Autodesk Fusion 360 part; units mm, degrees
note: some values were not read from the file. Set by a fixed rule: which sketch regions a step uses.
(part 3 of 3)
  circle A902 centre (-15.0186, -206.3325) radius 0.5023
  circle A903 centre (-15.0186, -209.9835) radius 0.5023
  circle A904 centre (-15.0186, -213.6344) radius 0.5023
  circle A905 centre (-15.0186, -217.2853) radius 0.5023
  circle A906 centre (-15.0186, -220.9363) radius 0.5023
  circle A907 centre (-15.0186, -224.5872) radius 0.5023
extrude "Estrusione56" cut sketch "Schizzo100" against normal blind 1 contours A0 | A1 | A2 | A3 | A4 | A5 | A6 | A7 | A8 | A9 | A10 | A11 | A12 | A13 | A14 | A15 | A16 | A17 | A18 | A19 | A20 | A21 | A22 | A23 | A24 | A25 | A26 | A27 | A28 | A29 | A30 | A31 | A32 | A33 | A34 | A35 | A36 | A37 | A38 | A39 | A40 | A41 | A42 | A43 | A44 | A45 | A46 | A47 | A48 | A49 | A50 | A51 | A52 | A53 | A54 | A55 | A56 | A57 | A58 | A59 | A60 | A61 | A62 | A63 | A64 | A65 | A66 | A67 | A68 | A69 | A70 | A71 | A72 | A73 | A74 | A75 | A76 | A77 | A78 | A79 | A80 | A81 | A82 | A83 | A84 | A85 | A86 | A87 | A88 | A89 | A90 | A91 | A92 | A93 | A94 | A95 | A96 | A97 | A98 | A99 | A100 | A101 | A102 | A103 | A104 | A105 | A106 | A107 | A108 | A109 | A110 | A111 | A112 | A113 | A114 | A115 | A116 | A117 | A118 | A119 | A120 | A121 | A122 | A123 | A124 | A125 | A126 | A127 | A128 | A129 | A130 | A131 | A132 | A133 | A134 | A135 | A136 | A137 | A138 | A139 | A140 | A141 | A142 | A143 | A144 | A145 | A146 | A147 | A148 | A149 | A150 | A151 | A152 | A153 | A154 | A155 | A156 | A157 | A158 | A159 | A160 | A161 | A162 | A163 | A164 | A165 | A166 | A167 | A168 | A169 | A170 | A171 | A172 | A173 | A174 | A175 | A176 | A177 | A178 | A179 | A180 | A181 | A182 | A183 | A184 | A185 | A186 | A187 | A188 | A189 | A190 | A191 | A192 | A193 | A194 | A195 | A196 | A197 | A198 | A199 | A200 | A201 | A202 | A203 | A204 | A205 | A206 | A207 | A208 | A209 | A210 | A211 | A212 | A213 | A214 | A215 | A216 | A217 | A218 | A219 | A220 | A221 | A222 | A223 | A224 | A225 | A226 | A227 | A228 | A229 | A230 | A231 | A232 | A233 | A234 | A235 | A236 | A237 | A238 | A239 | A240 | A241 | A242 | A243 | A244 | A245 | A246 | A247 | A248 | A249 | A250 | A251 | A252 | A253 | A254 | A255 | A256 | A257 | A258 | A259 | A260 | A261 | A262 | A263 | A264 | A265 | A266 | A267 | A268 | A269 | A270 | A271 | A272 | A273 | A274 | A275 | A276 | A277 | A278 | A279 | A280 | A281 | A282 | A283 | A284 | A285 | A286 | A287 | A288 | A289 | A290 | A291 | A292 | A293 | A294 | A295 | A296 | A297 | A298 | A299 | A300 | A301 | A302 | A303 | A304 | A305 | A306 | A307 | A308 | A309 | A310 | A311 | A312 | A313 | A314 | A315 | A316 | A317 | A318 | A319 | A320 | A321 | A322 | A323 | A324 | A325 | A326 | A327 | A328 | A329 | A330 | A331 | A332 | A333 | A334 | A335 | A336 | A337 | A338 | A339 | A340 | A341 | A342 | A343 | A344 | A345 | A346 | A347 | A348 | A349 | A350 | A351 | A352 | A353 | A354 | A355 | A356 | A357 | A358 | A359 | A360 | A361 | A362 | A363 | A364 | A365 | A366 | A367 | A368 | A369 | A370 | A371 | A372 | A373 | A374 | A375 | A376 | A377 | A378 | A379 | A380 | A381 | A382 | A383 | A384 | A385 | A386 | A387 | A388 | A389 | A390 | A391 | A392 | A393 | A394 | A395 | A396 | A397 | A398 | A399 | A400 | A401 | A402 | A403 | A404 | A405 | A406 | A407 | A408 | A409 | A410 | A411 | A412 | A413 | A414 | A415 | A416 | A417 | A418 | A419 | A420 | A421 | A422 | A423 | A424 | A425 | A426 | A427 | A428 | A429 | A430 | A431 | A432 | A433 | A434 | A435 | A436 | A437 | A438 | A439 | A440 | A441 | A442 | A443 | A444 | A445 | A446 | A447 | A448 | A449 | A450 | A451 | A452 | A453 | A454 | A455 | A456 | A457 | A458 | A459 | A460 | A461 | A462 | A463 | A464 | A465 | A466 | A467 | A468 | A469 | A470 | A471 | A472 | A473 | A474 | A475 | A476 | A477 | A478 | A479 | A480 | A481 | A482 | A483 | A484 | A485 | A486 | A487 | A488 | A489 | A490 | A491 | A492 | A493 | A494 | A495 | A496 | A497 | A498 | A499 | A500 | A501 | A502 | A503 | A504 | A505 | A506 | A507 | A508 | A509 | A510 | A511 | A512 | A513 | A514 | A515 | A516 | A517 | A518 | A519 | A520 | A521 | A522 | A523 | A524 | A525 | A526 | A527 | A528 | A529 | A530 | A531 | A532 | A533 | A534 | A535 | A536 | A537 | A538 | A539 | A540 | A541 | A542 | A543 | A544 | A545 | A546 | A547 | A548 | A549 | A550 | A551 | A552 | A553 | A554 | A555 | A556 | A557 | A558 | A559 | A560 | A561 | A562 | A563 | A564 | A565 | A566 | A567 | A568 | A569 | A570 | A571 | A572 | A573 | A574 | A575 | A576 | A577 | A578 | A579 | A580 | A581 | A582 | A583 | A584 | A585 | A586 | A587 | A588 | A589 | A590 | A591 | A592 | A593 | A594 | A595 | A596 | A597 | A598 | A599 | A600 | A601 | A602 | A603 | A604 | A605 | A606 | A607 | A608 | A609 | A610 | A611 | A612 | A613 | A614 | A615 | A616 | A617 | A618 | A619 | A620 | A621 | A622 | A623 | A624 | A625 | A626 | A627 | A628 | A629 | A630 | A631 | A632 | A633 | A634 | A635 | A636 | A637 | A638 | A639 | A640 | A641 | A642 | A643 | A644 | A645 | A646 | A647 | A648 | A649 | A650 | A651 | A652 | A653 | A654 | A655 | A656 | A657 | A658 | A659 | A660 | A661 | A662 | A663 | A664 | A665 | A666 | A667 | A668 | A669 | A670 | A671 | A672 | A673 | A674 | A675 | A676 | A677 | A678 | A679 | A680 | A681 | A682 | A683 | A684 | A685 | A686 | A687 | A688 | A689 | A690 | A691 | A692 | A693 | A694 | A695 | A696 | A697 | A698 | A699 | A700 | A701 | A702 | A703 | A704 | A705 | A706 | A707 | A708 | A709 | A710 | A711 | A712 | A713 | A714 | A715 | A716 | A717 | A718 | A719 | A720 | A721 | A722 | A723 | A724 | A725 | A726 | A727 | A728 | A729 | A730 | A731 | A732 | A733 | A734 | A735 | A736 | A737 | A738 | A739 | A740 | A741 | A742 | A743 | A744 | A745 | A746 | A747 | A748 | A749 | A750 | A751 | A752 | A753 | A754 | A755 | A756 | A757 | A758 | A759 | A760 | A761 | A762 | A763 | A764 | A765 | A766 | A767 | A768 | A769 | A770 | A771 | A772 | A773 | A774 | A775 | A776 | A777 | A778 | A779 | A780 | A781 | A782 | A783 | A784 | A785 | A786 | A787 | A788 | A789 | A790 | A791 | A792 | A793 | A794 | A795 | A796 | A797 | A798 | A799 | A800 | A801 | A802 | A803 | A804 | A805 | A806 | A807 | A808 | A809 | A810 | A811 | A812 | A813 | A814 | A815 | A816 | A817 | A818 | A819 | A820 | A821 | A822 | A823 | A824 | A825 | A826 | A827 | A828 | A829 | A830 | A831 | A832 | A833 | A834 | A835 | A836 | A837 | A838 | A839 | A840 | A841 | A842 | A843 | A844 | A845 | A846 | A847 | A848 | A849 | A850 | A851 | A852 | A853 | A854 | A855 | A856 | A857 | A858 | A859 | A860 | A861 | A862 | A863 | A864 | A865 | A866 | A867 | A868 | A869 | A870 | A871 | A872 | A873 | A874 | A875 | A876 | A877 | A878 | A879 | A880 | A881 | A882 | A883 | A884 | A885 | A886 | A887 | A888 | A889 | A890 | A891 | A892 | A893 | A894 | A895 | A896 | A897 | A898 | A899 | A900 | A901 | A902 | A903 | A904 | A905 | A906 | A907 picked at (15.0787, -5.3673) picked at (15.0787, -9.0183) picked at (15.0879, -12.8411) picked at (14.9196, -16.6361) picked at (14.8948, -20.2907) picked at (14.7587, -23.8997) picked at (14.8948, -27.5926) picked at (15.0731, -30.9982) picked at (15.3096, -34.6996) picked at (15.0912, -38.254) picked at (15.3096, -42.0014) picked at (15.3096, -45.6524) picked at (15.3096, -49.3033) picked at (15.3096, -52.9542) picked at (14.8814, -56.9112) picked at (15.3096, -60.2561) picked at (14.8709, -63.7829) picked at (14.6953, -67.6913) picked at (14.6953, -71.3423) picked at (14.6953, -74.9932) picked at (14.6953, -78.6441) picked at (15.0397, -82.3458) picked at (14.6953, -85.946) picked at (14.8598, -89.1907) picked at (14.6953, -93.2479) picked at (14.6953, -96.8988) picked at (14.6953, -100.5497) picked at (14.6953, -104.2007) picked at (15.0397, -107.9023) picked at (14.6953, -111.5026) picked at (14.7771, -115.1901) picked at (15.0397, -118.8551) picked at (15.0397, -122.506) picked at (15.0397, -126.157) picked at (15.1827, -129.532) picked at (15.1142, -133.1688) picked at (15.1142, -136.8198) picked at (15.0787, -140.4031) picked at (15.0787, -144.0541) picked at (15.0787, -147.705) picked at (15.1827, -151.4376) picked at (15.1827, -155.0886) picked at (15.1827, -158.7395) picked at (15.1827, -162.3904) picked at (15.1827, -166.0414) picked at (15.1827, -169.6923) picked at (15.1827, -173.3432) picked at (15.1827, -176.9942) picked at (15.1142, -180.631) picked at (15.1142, -184.2819) picked at (15.1142, -187.9329) picked at (15.0787, -191.5162) picked at (15.0787, -195.1672) picked at (15.0787, -198.8181) picked at (15.1827, -202.5507) picked at (15.1827, -206.2016) picked at (15.1827, -209.8526) picked at (15.1827, -213.5035) picked at (15.1827, -217.1544) picked at (15.1827, -220.8054) picked at (15.1827, -224.4563) picked at (13.2695, -7.1766) picked at (13.0358, -10.727) picked at (13.0358, -14.378) picked at (13.0575, -18.5125) picked at (13.0575, -22.1634) picked at (13.0856, -25.7509) picked at (13.0575, -29.4653) picked at (13.5004, -32.8578) picked at (13.2555, -36.4028) picked at (13.2555, -40.0538) picked at (13.2555, -43.7047) picked at (13.2555, -47.3556) picked at (13.5004, -51.1125) picked at (13.2555, -54.6575) picked at (13.0173, -58.3225) picked at (13.2555, -61.9594) picked at (13.1095, -65.5921) picked at (13.1095, -69.243) picked at (13.1095, -72.894) picked at (12.8861, -76.8024) picked at (13.1095, -80.1958) picked at (13.0505, -83.698) picked at (13.1095, -87.4977) picked at (13.1095, -91.1486) picked at (13.1095, -94.7996) picked at (13.1095, -98.4505) picked at (12.8861, -102.359) picked at (13.1095, -105.7524) picked at (13.0505, -109.2546) picked at (13.1095, -113.0542) picked at (13.1095, -116.7052) picked at (12.8861, -120.6137) picked at (12.8861, -124.2646) picked at (13.0084, -127.9155) picked at (13.2851, -131.3778) picked at (13.2851, -135.0288) picked at (13.305, -138.629) picked at (13.305, -142.2799) picked at (13.305, -145.9309) picked at (12.9495, -149.8407) picked at (12.9495, -153.4916) picked at (12.9495, -157.1426) picked at (12.9495, -160.7935) picked at (12.9495, -164.4444) picked at (12.9495, -168.0954) picked at (12.9495, -171.7463) picked at (12.9495, -175.3972) picked at (13.2851, -178.84) picked at (13.2851, -182.4909) picked at (13.2851, -186.1418) picked at (13.305, -189.7421) picked at (13.305, -193.393) picked at (12.9495, -197.3028) picked at (12.9495, -200.9538) picked at (12.9495, -204.6047) picked at (12.9495, -208.2557) picked at (12.9495, -211.9066) picked at (12.9495, -215.5575) picked at (12.9495, -219.2085) picked at (12.9495, -222.8594) picked at (10.7966, -5.3673) picked at (10.7966, -9.0183) picked at (10.8058, -12.8411) picked at (10.6375, -16.6361) picked at (10.6127, -20.2907) picked at (10.4766, -23.8997) picked at (10.6127, -27.5926) picked at (10.7911, -30.9982) picked at (11.0276, -34.6996) picked at (10.8091, -38.254) picked at (11.0276, -42.0014) picked at (11.0276, -45.6524) picked at (11.0276, -49.3033) picked at (11.0276, -52.9542) picked at (10.5993, -56.9112) picked at (11.0276, -60.2561) picked at (10.5888, -63.7829) picked at (10.4132, -67.6913) picked at (10.4132, -71.3423) picked at (10.4132, -74.9932) picked at (10.4132, -78.6441) picked at (10.7576, -82.3458) picked at (10.4132, -85.946) picked at (10.5777, -89.1907) picked at (10.4132, -93.2479) picked at (10.4132, -96.8988) picked at (10.4132, -100.5497) picked at (10.4132, -104.2007) picked at (10.7576, -107.9023) picked at (10.4132, -111.5026) picked at (10.495, -115.1901) picked at (10.7576, -118.8551) picked at (10.7576, -122.506) picked at (10.7576, -126.157) picked at (10.9006, -129.532) picked at (10.8321, -133.1688) picked at (10.8321, -136.8198) picked at (10.7966, -140.4031) picked at (10.7966, -144.0541) picked at (10.7966, -147.705) picked at (10.9006, -151.4376) picked at (10.9006, -155.0886) picked at (10.9006, -158.7395) picked at (10.9006, -162.3904) picked at (10.9006, -166.0414) picked at (10.9006, -169.6923) picked at (10.9006, -173.3432) picked at (10.9006, -176.9942) picked at (10.8321, -180.631) picked at (10.8321, -184.2819) picked at (10.8321, -187.9329) picked at (10.7966, -191.5162) picked at (10.7966, -195.1672) picked at (10.7966, -198.8181) picked at (10.9006, -202.5507) picked at (10.9006, -206.2016) picked at (10.9006, -209.8526) picked at (10.9006, -213.5035) picked at (10.9006, -217.1544) picked at (10.9006, -220.8054) picked at (10.9006, -224.4563) picked at (8.9874, -7.1766) picked at (8.9874, -10.8275) picked at (8.9874, -14.4784) picked at (8.8366, -18.5784) picked at (8.8366, -22.2293) picked at (8.8035, -25.7509) picked at (8.8366, -29.5312) picked at (8.7559, -33.0419) picked at (8.9258, -36.7037) picked at (8.9258, -40.3546) picked at (8.9258, -44.0056) picked at (8.9258, -47.6565) picked at (8.7559, -51.2966) picked at (8.9258, -54.9584) picked at (8.7353, -58.3225) picked at (8.9258, -62.2602) picked at (9.0124, -65.6414) picked at (9.0124, -69.2924) picked at (9.0124, -72.9433) picked at (8.604, -76.8024) picked at (9.0124, -80.2452) picked at (8.7684, -83.698) picked at (9.0124, -87.547) picked at (9.0124, -91.198) picked at (9.0124, -94.8489) picked at (9.0124, -98.4998) picked at (8.604, -102.359) picked at (9.0124, -105.8017) picked at (8.7684, -109.2546) picked at (9.0124, -113.1036) picked at (9.0124, -116.7545) picked at (8.604, -120.6137) picked at (8.604, -124.2646) picked at (8.7263, -127.9155) picked at (9.003, -131.3778) picked at (9.003, -135.0288) picked at (9.0229, -138.629) picked at (9.0229, -142.2799) picked at (9.0229, -145.9309) picked at (8.6674, -149.8407) picked at (8.6674, -153.4916) picked at (8.6674, -157.1426) picked at (8.6674, -160.7935) picked at (8.6674, -164.4444) picked at (8.6674, -168.0954) picked at (8.6674, -171.7463) picked at (8.6674, -175.3972) picked at (9.003, -178.84) picked at (9.003, -182.4909) picked at (9.003, -186.1418) picked at (9.0229, -189.7421) picked at (9.0229, -193.393) picked at (8.6674, -197.3028) picked at (8.6674, -200.9538) picked at (8.6674, -204.6047) picked at (8.6674, -208.2557) picked at (8.6674, -211.9066) picked at (8.6674, -215.5575) picked at (8.6674, -219.2085) picked at (8.6674, -222.8594) picked at (6.5499, -5.5067) picked at (6.5482, -9.1837) picked at (6.5501, -12.955) picked at (6.3554, -16.6361) picked at (6.3306, -20.2907) picked at (6.5891, -23.6719) picked at (6.3306, -27.5926) picked at (6.5201, -31.0481) picked at (6.7455, -34.7777) picked at (6.5427, -38.4622) picked at (6.7455, -42.0795) picked at (6.7455, -45.7305) picked at (6.7455, -49.3814) picked at (6.7455, -53.0323) picked at (6.5482, -56.6459) picked at (6.7455, -60.3342) picked at (6.453, -64.1019) picked at (6.6525, -67.5027) picked at (6.6525, -71.1536) picked at (6.6525, -74.8046) picked at (6.6525, -78.4555) picked at (6.3081, -82.0558) picked at (6.6525, -85.7574) picked at (6.2956, -89.1907) picked at (6.6525, -93.0592) picked at (6.6525, -96.7102) picked at (6.6525, -100.3611) picked at (6.6525, -104.0121) picked at (6.3081, -107.6123) picked at (6.6525, -111.3139) picked at (6.5891, -114.9453) picked at (6.3081, -118.5651) picked at (6.3081, -122.216) picked at (6.3081, -125.867) picked at (6.1651, -129.7938) picked at (6.2336, -133.4588) picked at (6.2336, -137.1098) picked at (6.2691, -140.8283) picked at (6.2691, -144.4792) picked at (6.2691, -148.1302) picked at (6.1651, -151.6994) picked at (6.6185, -155.0886) picked at (6.1651, -159.0013) picked at (6.1651, -162.6522) picked at (6.1651, -166.3032) picked at (6.6185, -169.6923) picked at (6.1651, -173.605) picked at (6.6185, -176.9942) picked at (6.2336, -180.921) picked at (6.2336, -184.5719) picked at (6.2336, -188.2229) picked at (6.2691, -191.9414) picked at (6.2691, -195.5923) picked at (6.2691, -199.2433) picked at (6.1651, -202.8125) picked at (6.1651, -206.4634) picked at (6.1651, -210.1144) picked at (6.1651, -213.7653) picked at (6.1651, -217.4163) picked at (6.1651, -221.0672) picked at (6.1651, -224.7181) picked at (4.7142, -7.5905) picked at (4.5486, -11.2664) picked at (4.5486, -14.9173) picked at (4.5361, -18.5466) picked at (4.5361, -22.1975) picked at (4.4728, -25.4281) picked at (4.5361, -29.4994) picked at (4.4532, -33.0278) picked at (4.4026, -36.3809) picked at (4.6913, -40.0538) picked at (4.4026, -43.6827) picked at (4.6913, -47.3556) picked at (4.4532, -51.2825) picked at (4.6913, -54.6575) picked at (4.5701, -58.3586) picked at (4.6913, -61.9594) picked at (4.4348, -65.8692) picked at (4.4348, -69.5201) picked at (4.4348, -73.1711) picked at (4.8433, -76.6138) picked at (4.4348, -80.4729) picked at (4.4864, -83.698) picked at (4.4348, -87.7748) picked at (4.4348, -91.4257) picked at (4.4348, -95.0767) picked at (4.4348, -98.7276) picked at (4.8433, -102.1703) picked at (4.4348, -106.0295) picked at (4.4864, -109.2546) picked at (4.4348, -113.3313) picked at (4.4348, -116.9823) picked at (4.8433, -120.425) picked at (4.8433, -124.076) picked at (4.75, -128.0098) picked at (4.4442, -131.5665) picked at (4.4442, -135.2174) picked at (4.4244, -138.919) picked at (4.4244, -142.5699) picked at (4.4244, -146.2209) picked at (4.7798, -149.6129) picked at (4.7798, -153.2639) picked at (4.7798, -156.9148) picked at (4.7798, -160.5657) picked at (4.7798, -164.2167) picked at (4.7798, -167.8676) picked at (4.7798, -171.5185) picked at (4.7798, -175.1695) picked at (4.4442, -179.0286) picked at (4.4442, -182.6795) picked at (4.4442, -186.3305) picked at (4.4244, -190.0321) picked at (4.4244, -193.683) picked at (4.7798, -197.0751) picked at (4.7798, -200.726) picked at (4.7798, -204.377) picked at (4.7798, -208.0279) picked at (4.7798, -211.6788) picked at (4.7798, -215.3298) picked at (4.7798, -218.9807) picked at (4.7798, -222.6316) picked at (2.0725, -5.6944) picked at (2.2325, -9.3799) picked at (2.2697, -12.7836) picked at (2.0972, -16.3244) picked at (2.3548, -20.021) picked at (2.3548, -23.6719) picked at (2.3548, -27.3229) picked at (2.0053, -30.9908) picked at (2.001, -34.8836) picked at (2.2499, -38.3202) picked at (2.001, -42.1855) picked at (2.001, -45.8364) picked at (1.9091, -49.4952) picked at (1.9091, -53.1461) picked at (1.9464, -56.5499) picked at (2.001, -60.4401) picked at (2.0486, -63.7902) picked at (2.3704, -67.5027) picked at (2.3704, -71.1536) picked at (2.3704, -74.8046) picked at (2.3704, -78.4555) picked at (2.026, -82.0558) picked at (2.3704, -85.7574) picked at (2.0135, -89.1907) picked at (2.3704, -93.0592) picked at (2.3704, -96.7102) picked at (2.3704, -100.3611) picked at (2.3704, -104.0121) picked at (2.026, -107.6123) picked at (2.3704, -111.3139) picked at (2.307, -114.9453) picked at (2.026, -118.5651) picked at (2.026, -122.216) picked at (2.026, -125.867) picked at (2.3365, -129.532) picked at (2.268, -133.1688) picked at (2.268, -136.8198) picked at (2.2325, -140.4031) picked at (2.2325, -144.0541) picked at (2.2325, -147.705) picked at (2.3365, -151.4376) picked at (2.3365, -155.0886) picked at (2.3365, -158.7395) picked at (2.3365, -162.3904) picked at (2.3365, -166.0414) picked at (2.3365, -169.6923) picked at (2.3365, -173.3432) picked at (2.3365, -176.9942) picked at (2.268, -180.631) picked at (2.268, -184.2819) picked at (2.268, -187.9329) picked at (2.2325, -191.5162) picked at (2.2325, -195.1672) picked at (2.2325, -198.8181) picked at (2.3365, -202.5507) picked at (2.3365, -206.2016) picked at (2.3365, -209.8526) picked at (2.3365, -213.5035) picked at (2.3365, -217.1544) picked at (2.3365, -220.8054) picked at (2.3365, -224.4563) picked at (0.2783, -7.2156) picked at (0.2632, -10.8281) picked at (0.2632, -14.479) picked at (0.1456, -18.1262) picked at (0.1456, -21.7771) picked at (0.1478, -25.6427) picked at (0.1456, -29.079) picked at (0.4388, -32.8525) picked at (0.1961, -36.4169) picked at (0.1961, -40.0679) picked at (0.1961, -43.7188) picked at (0.1961, -47.3697) picked at (0.4388, -51.1072) picked at (0.1961, -54.6716) picked at (0.4588, -58.5754) picked at (0.1961, -61.9735) picked at (0.2043, -65.4434) picked at (0.2043, -69.0943) picked at (0.2043, -72.7452) picked at (0.4977, -76.5942) picked at (0.2043, -80.0471) picked at (0.4049, -83.8791) picked at (0.2043, -87.349) picked at (0.2043, -90.9999) picked at (0.2043, -94.6508) picked at (0.2043, -98.3018) picked at (0.4977, -102.1508) picked at (0.2043, -105.6036) picked at (0.4049, -109.4356) picked at (0.2043, -112.9055) picked at (0.2043, -116.5564) picked at (0.4977, -120.4055) picked at (0.4977, -124.0564) picked at (0.0793, -127.9425) picked at (0.4977, -131.3583) picked at (0.4977, -135.0092) picked at (0.5272, -138.6431) picked at (0.5272, -142.294) picked at (0.5272, -145.945) picked at (-0.0178, -149.7995) picked at (-0.0178, -153.4504) picked at (-0.0178, -157.1013) picked at (-0.0178, -160.7523) picked at (-0.0178, -164.4032) picked at (-0.0178, -168.0541) picked at (-0.0178, -171.7051) picked at (-0.0178, -175.356) picked at (0.4977, -178.8204) picked at (0.4977, -182.4713) picked at (0.4977, -186.1223) picked at (0.5272, -189.7562) picked at (0.5272, -193.4071) picked at (-0.0178, -197.2616) picked at (-0.0178, -200.9125) picked at (-0.0178, -204.5635) picked at (-0.0178, -208.2144) picked at (-0.0178, -211.8654) picked at (-0.0178, -215.5163) picked at (-0.0178, -219.1672) picked at (-0.0178, -222.8182) picked at (-2.2096, -5.6944) picked at (-2.1913, -9.0358) picked at (-2.0141, -12.955) picked at (-2.1849, -16.3244) picked at (-1.9273, -20.021) picked at (-1.9273, -23.6719) picked at (-1.9273, -27.3229) picked at (-2.2768, -30.9908) picked at (-2.0636, -34.5936) picked at (-2.3379, -38.2259) picked at (-2.0636, -41.8955) picked at (-2.0636, -45.5464) picked at (-2.373, -49.4952) picked at (-2.373, -53.1461) picked at (-2.2561, -56.7892) picked at (-2.0636, -60.1502) picked at (-2.2335, -63.7902) picked at (-2.4556, -67.6805) picked at (-2.4556, -71.3314) picked at (-2.4556, -74.9823) picked at (-2.4556, -78.6333) picked at (-2.2561, -82.0558) picked at (-2.4556, -85.9352) picked at (-2.0068, -89.7162) picked at (-2.4556, -93.237) picked at (-2.4556, -96.888) picked at (-2.4556, -100.5389) picked at (-2.4556, -104.1898) picked at (-2.2561, -107.6123) picked at (-2.4556, -111.4917) picked at (-1.9751, -114.9453) picked at (-2.2561, -118.5651) picked at (-2.2561, -122.216) picked at (-2.2561, -125.867) picked at (-1.9456, -129.532) picked at (-2.0141, -133.1688) picked at (-2.0141, -136.8198) picked at (-2.2951, -140.8283) picked at (-2.2951, -144.4792) picked at (-2.2951, -148.1302) picked at (-1.9456, -151.4376) picked at (-1.9456, -155.0886) picked at (-1.9456, -158.7395) picked at (-1.9456, -162.3904) picked at (-1.9456, -166.0414) picked at (-1.9456, -169.6923) picked at (-1.9456, -173.3432) picked at (-1.9456, -176.9942) picked at (-2.0141, -180.631) picked at (-2.0141, -184.2819) picked at (-2.0141, -187.9329) picked at (-2.2951, -191.9414) picked at (-2.2951, -195.5923) picked at (-2.2951, -199.2433) picked at (-1.9456, -202.5507) picked at (-1.9456, -206.2016) picked at (-1.9456, -209.8526) picked at (-1.9456, -213.5035) picked at (-1.9456, -217.1544) picked at (-1.9456, -220.8054) picked at (-1.9456, -224.4563) picked at (-3.8441, -7.5019) picked at (-4.1232, -11.0577) picked at (-4.1232, -14.7086) picked at (-4.0914, -18.1262) picked at (-4.0914, -21.7771) picked at (-3.8589, -25.743) picked at (-4.0914, -29.079) picked at (-3.8307, -32.9695) picked at (-4.1822, -36.7007) picked at (-4.0903, -40.3438) picked at (-4.1822, -44.0026) picked at (-4.0903, -47.6456) picked at (-3.8307, -51.2242) picked at (-4.0903, -54.9475) picked at (-3.8451, -58.3342) picked at (-4.0903, -62.2494) picked at (-4.0914, -65.5884) picked at (-4.0914, -69.2393) picked at (-4.0914, -72.8902) picked at (-4.0653, -76.5631) picked at (-4.0914, -80.1921) picked at (-3.7843, -83.8961) picked at (-4.0914, -87.494) picked at (-4.0914, -91.1449) picked at (-4.0914, -94.7958) picked at (-4.0914, -98.4468) picked at (-4.0653, -102.1197) picked at (-4.0914, -105.7486) picked at (-3.7843, -109.4527) picked at (-4.0914, -113.0505) picked at (-4.0914, -116.7014) picked at (-4.0653, -120.3743) picked at (-4.0653, -124.0253) picked at (-3.9941, -127.7995) picked at (-3.8234, -131.3271) picked at (-3.8234, -134.9781) picked at (-4.1043, -138.9866) picked at (-4.1043, -142.6375) picked at (-4.1043, -146.2885) picked at (-4.2083, -149.8577) picked at (-4.2083, -153.5087) picked at (-4.2083, -157.1596) picked at (-4.2083, -160.8105) picked at (-4.2083, -164.4615) picked at (-4.2083, -168.1124) picked at (-4.2083, -171.7633) picked at (-4.2083, -175.4143) picked at (-3.8234, -178.7893) picked at (-3.8234, -182.4402) picked at (-3.8234, -186.0912) picked at (-4.1043, -190.0997) picked at (-4.1043, -193.7506) picked at (-4.2083, -197.3199) picked at (-4.2083, -200.9708) picked at (-4.2083, -204.6217) picked at (-4.2083, -208.2727) picked at (-4.2083, -211.9236) picked at (-4.2083, -215.5745) picked at (-4.2083, -219.2255) picked at (-4.2083, -222.8764) picked at (-6.2963, -5.5067) picked at (-6.298, -9.1837) picked at (-6.2962, -12.955) picked at (-6.4909, -16.6361) picked at (-6.5156, -20.2907) picked at (-6.2572, -23.6719) picked at (-6.5156, -27.5926) picked at (-6.3261, -31.0481) picked at (-6.1008, -34.7777) picked at (-6.3036, -38.4622) picked at (-6.1008, -42.0795) picked at (-6.1008, -45.7305) picked at (-6.1008, -49.3814) picked at (-6.1008, -53.0323) picked at (-6.298, -56.6459) picked at (-6.1008, -60.3342) picked at (-6.3933, -64.1019) picked at (-6.1938, -67.5027) picked at (-6.1938, -71.1536) picked at (-6.1938, -74.8046) picked at (-6.1938, -78.4555) picked at (-6.5382, -82.0558) picked at (-6.1938, -85.7574) picked at (-6.5507, -89.1907) picked at (-6.1938, -93.0592) picked at (-6.1938, -96.7102) picked at (-6.1938, -100.3611) picked at (-6.1938, -104.0121) picked at (-6.5382, -107.6123) picked at (-6.1938, -111.3139) picked at (-6.2572, -114.9453) picked at (-6.5382, -118.5651) picked at (-6.5382, -122.216) picked at (-6.5382, -125.867) picked at (-6.6812, -129.7938) picked at (-6.6127, -133.4588) picked at (-6.6127, -137.1098) picked at (-6.5772, -140.8283) picked at (-6.5772, -144.4792) picked at (-6.5772, -148.1302) picked at (-6.6812, -151.6994) picked at (-6.2277, -155.0886) picked at (-6.6812, -159.0013) picked at (-6.6812, -162.6522) picked at (-6.6812, -166.3032) picked at (-6.2277, -169.6923) picked at (-6.6812, -173.605) picked at (-6.2277, -176.9942) picked at (-6.6127, -180.921) picked at (-6.6127, -184.5719) picked at (-6.6127, -188.2229) picked at (-6.5772, -191.9414) picked at (-6.5772, -195.5923) picked at (-6.5772, -199.2433) picked at (-6.6812, -202.8125) picked at (-6.6812, -206.4634) picked at (-6.6812, -210.1144) picked at (-6.6812, -213.7653) picked at (-6.6812, -217.4163) picked at (-6.6812, -221.0672) picked at (-6.6812, -224.7181) picked at (-8.3864, -7.5041) picked at (-8.1128, -10.9686) picked at (-8.1128, -14.6195) picked at (-8.3248, -18.449) picked at (-8.3248, -22.0999) picked at (-8.1409, -25.5311) picked at (-8.3248, -29.4018) picked at (-8.1128, -32.8742) picked at (-7.91, -36.5869) picked at (-7.91, -40.2378) picked at (-7.91, -43.8888) picked at (-7.91, -47.5397) picked at (-8.1128, -51.1288) picked at (-7.91, -54.8416) picked at (-8.402, -58.5044) picked at (-7.91, -62.1434) picked at (-8.5244, -65.8496) picked at (-8.5244, -69.5006) picked at (-8.5244, -73.1515) picked at (-8.18, -76.8531) picked at (-8.5244, -80.4534) picked at (-8.0664, -83.8961) picked at (-8.5244, -87.7552) picked at (-8.5244, -91.4062) picked at (-8.5244, -95.0571) picked at (-8.5244, -98.708) picked at (-8.18, -102.4097) picked at (-8.5244, -106.0099) picked at (-8.0664, -109.4527) picked at (-8.5244, -113.3118) picked at (-8.5244, -116.9627) picked at (-8.18, -120.6643) picked at (-8.18, -124.3153) picked at (-8.4518, -127.7306) picked at (-8.1054, -131.3271) picked at (-8.1054, -134.9781) picked at (-8.3864, -138.9866) picked at (-8.3864, -142.6375) picked at (-8.3864, -146.2885) picked at (-8.0369, -149.5959) picked at (-8.0369, -153.2468) picked at (-8.4904, -157.1596) picked at (-8.4904, -160.8105) picked at (-8.4904, -164.4615) picked at (-8.0369, -167.8506) picked at (-8.4904, -171.7633) picked at (-8.0369, -175.1525) picked at (-8.1054, -178.7893) picked at (-8.1054, -182.4402) picked at (-8.1054, -186.0912) picked at (-8.3864, -190.0997) picked at (-8.3864, -193.7506) picked at (-8.0369, -197.0581) picked at (-8.4904, -200.9708) picked at (-8.4904, -204.6217) picked at (-8.4904, -208.2727) picked at (-8.4904, -211.9236) picked at (-8.4904, -215.5745) picked at (-8.4904, -219.2255) picked at (-8.4904, -222.8764) picked at (-10.6138, -5.3673) picked at (-10.6138, -9.0183) picked at (-10.5765, -12.8823) picked at (-10.773, -16.6361) picked at (-10.7977, -20.2907) picked at (-10.9338, -23.8997) picked at (-10.7977, -27.5926) picked at (-10.6194, -30.9982) picked at (-10.8453, -34.8836) picked at (-10.8749, -38.2952) picked at (-10.8453, -42.1855) picked at (-10.8453, -45.8364) picked at (-10.6278, -49.1973) picked at (-10.6278, -52.8483) picked at (-10.8111, -56.9112) picked at (-10.8453, -60.4401) picked at (-10.8216, -63.7829) picked at (-10.9972, -67.6913) picked at (-10.9972, -71.3423) picked at (-10.9972, -74.9932) picked at (-10.9972, -78.6441) picked at (-10.6528, -82.3458) picked at (-10.9972, -85.946) picked at (-10.8328, -89.1907) picked at (-10.9972, -93.2479) picked at (-10.9972, -96.8988) picked at (-10.9972, -100.5497) picked at (-10.9972, -104.2007) picked at (-10.6528, -107.9023) picked at (-10.9972, -111.5026) picked at (-10.9154, -115.1901) picked at (-10.6528, -118.8551) picked at (-10.6528, -122.506) picked at (-10.6528, -126.157) picked at (-10.5098, -129.532) picked at (-10.5783, -133.1688) picked at (-10.5783, -136.8198) picked at (-10.8593, -140.8283) picked at (-10.8593, -144.4792) picked at (-10.8593, -148.1302) picked at (-10.5098, -151.4376) picked at (-10.5098, -155.0886) picked at (-10.5098, -158.7395) picked at (-10.5098, -162.3904) picked at (-10.5098, -166.0414) picked at (-10.5098, -169.6923) picked at (-10.5098, -173.3432) picked at (-10.5098, -176.9942) picked at (-10.5783, -180.631) picked at (-10.5783, -184.2819) picked at (-10.5783, -187.9329) picked at (-10.8593, -191.9414) picked at (-10.8593, -195.5923) picked at (-10.8593, -199.2433) picked at (-10.5098, -202.5507) picked at (-10.5098, -206.2016) picked at (-10.5098, -209.8526) picked at (-10.5098, -213.5035) picked at (-10.5098, -217.1544) picked at (-10.5098, -220.8054) picked at (-10.5098, -224.4563) picked at (-12.423, -7.1766) picked at (-12.423, -10.8275) picked at (-12.423, -14.4784) picked at (-12.6069, -18.449) picked at (-12.6069, -22.0999) picked at (-12.4286, -25.5055) picked at (-12.6069, -29.4018) picked at (-12.6203, -33.1639) picked at (-12.1921, -36.5088) picked at (-12.1921, -40.1597) picked at (-12.1921, -43.8107) picked at (-12.1921, -47.4616) picked at (-12.6203, -51.4186) picked at (-12.1921, -54.7635) picked at (-12.4105, -58.3179) picked at (-12.1921, -62.0653) picked at (-12.8064, -65.8496) picked at (-12.8064, -69.5006) picked at (-12.8064, -73.1515) picked at (-12.462, -76.8531) picked at (-12.8064, -80.4534) picked at (-12.7247, -84.1409) picked at (-12.8064, -87.7552) picked at (-12.8064, -91.4062) picked at (-12.8064, -95.0571) picked at (-12.8064, -98.708) picked at (-12.462, -102.4097) picked at (-12.8064, -106.0099) picked at (-12.7247, -109.6974) picked at (-12.8064, -113.3118) picked at (-12.8064, -116.9627) picked at (-12.462, -120.6643) picked at (-12.462, -124.3153) picked at (-12.6198, -127.7184) picked at (-12.3875, -131.3271) picked at (-12.3875, -134.9781) picked at (-12.423, -138.5614) picked at (-12.423, -142.2124) picked at (-12.423, -145.8633) picked at (-12.319, -149.5959) picked at (-12.319, -153.2468) picked at (-12.319, -156.8978) picked at (-12.319, -160.5487) picked at (-12.319, -164.1997) picked at (-12.319, -167.8506) picked at (-12.319, -171.5015) picked at (-12.319, -175.1525) picked at (-12.3875, -178.7893) picked at (-12.3875, -182.4402) picked at (-12.3875, -186.0912) picked at (-12.423, -189.6745) picked at (-12.423, -193.3255) picked at (-12.319, -197.0581) picked at (-12.319, -200.709) picked at (-12.319, -204.3599) picked at (-12.319, -208.0109) picked at (-12.319, -211.6618) picked at (-12.319, -215.3127) picked at (-12.319, -218.9637) picked at (-12.319, -222.6146) picked at (-14.8959, -5.3673) picked at (-14.8959, -9.0183) picked at (-14.8586, -12.8823) picked at (-15.055, -16.6361) picked at (-15.0798, -20.2907) picked at (-15.2159, -23.8997) picked at (-15.0798, -27.5926) picked at (-14.9015, -30.9982) picked at (-15.1274, -34.8836) picked at (-15.157, -38.2952) picked at (-15.1274, -42.1855) picked at (-15.1274, -45.8364) picked at (-14.9099, -49.1973) picked at (-14.9099, -52.8483) picked at (-15.0932, -56.9112) picked at (-15.1274, -60.4401) picked at (-15.1037, -63.7829) picked at (-15.2793, -67.6913) picked at (-15.2793, -71.3423) picked at (-15.2793, -74.9932) picked at (-15.2793, -78.6441) picked at (-14.9349, -82.3458) picked at (-15.2793, -85.946) picked at (-15.1148, -89.1907) picked at (-15.2793, -93.2479) picked at (-15.2793, -96.8988) picked at (-15.2793, -100.5497) picked at (-15.2793, -104.2007) picked at (-14.9349, -107.9023) picked at (-15.2793, -111.5026) picked at (-15.1975, -115.1901) picked at (-14.9349, -118.8551) picked at (-14.9349, -122.506) picked at (-14.9349, -126.157) picked at (-14.7919, -129.532) picked at (-14.8604, -133.1688) picked at (-14.8604, -136.8198) picked at (-15.1414, -140.8283) picked at (-15.1414, -144.4792) picked at (-15.1414, -148.1302) picked at (-14.7919, -151.4376) picked at (-14.7919, -155.0886) picked at (-14.7919, -158.7395) picked at (-14.7919, -162.3904) picked at (-14.7919, -166.0414) picked at (-14.7919, -169.6923) picked at (-14.7919, -173.3432) picked at (-14.7919, -176.9942) picked at (-14.8604, -180.631) picked at (-14.8604, -184.2819) picked at (-14.8604, -187.9329) picked at (-15.1414, -191.9414) picked at (-15.1414, -195.5923) picked at (-15.1414, -199.2433) picked at (-14.7919, -202.5507) picked at (-14.7919, -206.2016) picked at (-14.7919, -209.8526) picked at (-14.7919, -213.5035) picked at (-14.7919, -217.1544) picked at (-14.7919, -220.8054) picked at (-14.7919, -224.4563) bodies 6
move_body "Sposta17" [rolled back]
move_body "Sposta18" [rolled back]
move_body "Sposta14" [suppressed]
move_body "Sposta15" [suppressed]
move_body "Sposta16" [suppressed]
